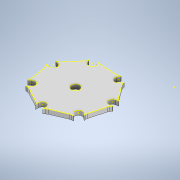
# Autodesk Inventor part: sprocket7_mk2
Saved by Autodesk Inventor 2020 (Build 240168000, 168)
## iProperties
Created: 2019-07-16
Part Number: sprocket7_mk2
Material: Generic
Document SubType Name: Modeling
Designer: erwin
Density: 1 g/cm^3
Appearance: Default
Author: erwin
Autodesk Inventor part; units mm, degrees
ref_plane "YZ Plane" through (0, 0, 0) normal (1, 0, 0) x (0, 1, 0)
ref_plane "XZ Plane" through (0, 0, 0) normal (0, 1, 0) x (-1, 0, 0)
ref_plane "XY Plane" through (0, 0, 0) normal (0, 0, 1) x (1, 0, 0)
sketch "Sketch2" plane through (0, 0, 0) normal (0, 1, 0) x (-1, 0, 0)
  line L0 (77.8598, 129.5505) -> (181.2412, 129.5505)
  line L1 (129.5505, 77.8598) -> (129.5505, 181.2412)
  line L2 (208.1814, 165.1629) -> (207.9893, 170.0518)
  line L3 (207.9893, 170.0518) -> (209.1581, 174.8028)
  line L4 (209.1581, 174.8028) -> (211.5965, 179.0445)
  line L5 (211.5965, 179.0445) -> (215.1139, 182.4454)
  line L6 (215.1139, 182.4454) -> (217.4859, 184.4007)
  line L7 (217.4859, 184.4007) -> (218.8706, 185.7147)
  line L8 (218.8706, 185.7147) -> (219.868, 187.3423)
  line L9 (219.868, 187.3423) -> (220.4102, 189.1727)
  line L10 (220.4102, 189.1727) -> (220.4602, 191.0809)
  line L11 (220.4602, 191.0809) -> (220.0145, 192.9371)
  line L12 (220.0145, 192.9371) -> (219.1037, 194.6147)
  line L13 (219.1037, 194.6147) -> (217.7897, 195.9994)
  line L14 (217.7897, 195.9994) -> (216.162, 196.9968)
  line L15 (216.162, 196.9968) -> (214.3317, 197.5389)
  line L16 (214.3317, 197.5389) -> (212.4235, 197.5889)
  line L17 (212.4235, 197.5889) -> (210.5673, 197.1433)
  line L18 (210.5673, 197.1433) -> (208.8897, 196.2324)
  line L19 (208.8897, 196.2324) -> (206.2971, 194.5807)
  line L20 (206.2971, 194.5807) -> (201.9757, 192.2864)
  line L21 (201.9757, 192.2864) -> (197.1881, 191.2781)
  line L22 (197.1881, 191.2781) -> (192.3084, 191.6346)
  line L23 (192.3084, 191.6346) -> (187.7182, 193.3281)
  line L24 (187.7182, 193.3281) -> (150.7331, 213.2305)
  line L25 (150.7331, 213.2305) -> (146.7911, 216.1285)
  line L26 (146.7911, 216.1285) -> (143.8054, 220.0046)
  line L27 (143.8054, 220.0046) -> (142.0094, 224.5557)
  line L28 (142.0094, 224.5557) -> (141.5435, 229.4261)
  line L29 (141.5435, 229.4261) -> (141.4937, 232.4997)
  line L30 (141.4937, 232.4997) -> (141.3297, 234.4016)
  line L31 (141.3297, 234.4016) -> (140.6791, 236.1962)
  line L32 (140.6791, 236.1962) -> (139.5861, 237.7613)
  line L33 (139.5861, 237.7613) -> (138.1253, 238.9901)
  line L34 (138.1253, 238.9901) -> (136.3963, 239.799)
  line L35 (136.3963, 239.799) -> (134.5168, 240.1329)
  line L36 (134.5168, 240.1329) -> (132.6149, 239.9689)
  line L37 (132.6149, 239.9689) -> (130.8203, 239.3182)
  line L38 (130.8203, 239.3182) -> (129.2552, 238.2252)
  line L39 (129.2552, 238.2252) -> (128.0264, 236.7645)
  line L40 (128.0264, 236.7645) -> (127.2175, 235.0354)
  line L41 (127.2175, 235.0354) -> (126.8836, 233.1559)
  line L42 (126.8836, 233.1559) -> (126.5586, 230.0991)
  line L43 (126.5586, 230.0991) -> (125.658, 225.29)
  line L44 (125.658, 225.29) -> (123.4612, 220.9182)
  line L45 (123.4612, 220.9182) -> (120.1401, 217.3254)
  line L46 (120.1401, 217.3254) -> (115.9541, 214.7925)
  line L47 (115.9541, 214.7925) -> (77.334, 198.2854)
  line L48 (77.334, 198.2854) -> (72.6104, 197.0103)
  line L49 (72.6104, 197.0103) -> (67.7184, 197.0926)
  line L50 (67.7184, 197.0926) -> (63.0404, 198.526)
  line L51 (63.0404, 198.526) -> (58.9421, 201.1984)
  line L52 (58.9421, 201.1984) -> (56.508, 203.0759)
  line L53 (56.508, 203.0759) -> (54.9188, 204.1335)
  line L54 (54.9188, 204.1335) -> (53.1101, 204.7437)
  line L55 (53.1101, 204.7437) -> (51.205, 204.865)
  line L56 (51.205, 204.865) -> (49.3334, 204.4891)
  line L57 (49.3334, 204.4891) -> (47.623, 203.6416)
  line L58 (47.623, 203.6416) -> (46.1901, 202.3802)
  line L59 (46.1901, 202.3802) -> (45.1326, 200.7911)
  line L60 (45.1326, 200.7911) -> (44.5223, 198.9823)
  line L61 (44.5223, 198.9823) -> (44.401, 197.0772)
  line L62 (44.401, 197.0772) -> (44.777, 195.2057)
  line L63 (44.777, 195.2057) -> (45.6245, 193.4952)
  line L64 (45.6245, 193.4952) -> (46.8858, 192.0624)
  line L65 (46.8858, 192.0624) -> (49.073, 189.9023)
  line L66 (49.073, 189.9023) -> (52.2714, 186.1998)
  line L67 (52.2714, 186.1998) -> (54.3197, 181.7566)
  line L68 (54.3197, 181.7566) -> (55.058, 176.9199)
  line L69 (55.058, 176.9199) -> (54.4284, 172.0679)
  line L70 (54.4284, 172.0679) -> (43.2549, 131.5815)
  line L71 (43.2549, 131.5815) -> (41.3067, 127.0934)
  line L72 (41.3067, 127.0934) -> (38.1923, 123.3201)
  line L73 (38.1923, 123.3201) -> (34.1549, 120.5564)
  line L74 (34.1549, 120.5564) -> (29.5103, 119.0184)
  line L75 (29.5103, 119.0184) -> (26.5248, 118.2859)
  line L76 (26.5248, 118.2859) -> (24.7071, 117.7028)
  line L77 (24.7071, 117.7028) -> (23.1023, 116.6692)
  line L78 (23.1023, 116.6692) -> (21.8196, 115.2553)
  line L79 (21.8196, 115.2553) -> (20.9467, 113.5577)
  line L80 (20.9467, 113.5577) -> (20.5428, 111.692)
  line L81 (20.5428, 111.692) -> (20.6356, 109.7853)
  line L82 (20.6356, 109.7853) -> (21.2187, 107.9677)
  line L83 (21.2187, 107.9677) -> (22.2523, 106.3628)
  line L84 (22.2523, 106.3628) -> (23.6661, 105.0802)
  line L85 (23.6661, 105.0802) -> (25.3638, 104.2072)
  line L86 (25.3638, 104.2072) -> (27.2295, 103.8034)
  line L87 (27.2295, 103.8034) -> (29.1361, 103.8961)
  line L88 (29.1361, 103.8961) -> (32.1886, 104.2594)
  line L89 (32.1886, 104.2594) -> (37.0775, 104.4515)
  line L90 (37.0775, 104.4515) -> (41.8285, 103.2827)
  line L91 (41.8285, 103.2827) -> (46.0703, 100.8443)
  line L92 (46.0703, 100.8443) -> (49.4712, 97.3269)
  line L93 (49.4712, 97.3269) -> (74.1582, 63.3482)
  line L94 (74.1582, 63.3482) -> (76.4524, 59.0268)
  line L95 (76.4524, 59.0268) -> (77.4607, 54.2392)
  line L96 (77.4607, 54.2392) -> (77.1042, 49.3595)
  line L97 (77.1042, 49.3595) -> (75.4108, 44.7692)
  line L98 (75.4108, 44.7692) -> (74.122, 41.9784)
  line L99 (74.122, 41.9784) -> (73.4446, 40.1937)
  line L100 (73.4446, 40.1937) -> (73.2521, 38.2945)
  line L101 (73.2521, 38.2945) -> (73.5578, 36.4102)
  line L102 (73.5578, 36.4102) -> (74.3407, 34.6693)
  line L103 (74.3407, 34.6693) -> (75.5476, 33.1902)
  line L104 (75.5476, 33.1902) -> (77.0961, 32.074)
  line L105 (77.0961, 32.074) -> (78.8808, 31.3966)
  line L106 (78.8808, 31.3966) -> (80.78, 31.2041)
  line L107 (80.78, 31.2041) -> (82.6643, 31.5098)
  line L108 (82.6643, 31.5098) -> (84.4053, 32.2927)
  line L109 (84.4053, 32.2927) -> (85.8843, 33.4996)
  line L110 (85.8843, 33.4996) -> (87.0006, 35.0481)
  line L111 (87.0006, 35.0481) -> (88.6197, 37.6612)
  line L112 (88.6197, 37.6612) -> (91.5177, 41.6033)
  line L113 (91.5177, 41.6033) -> (95.3937, 44.589)
  line L114 (95.3937, 44.589) -> (99.9449, 46.385)
  line L115 (99.9449, 46.385) -> (104.8153, 46.8509)
  line L116 (104.8153, 46.8509) -> (146.773, 44.9666)
  line L117 (146.773, 44.9666) -> (151.582, 44.066)
  line L118 (151.582, 44.066) -> (155.9538, 41.8692)
  line L119 (155.9538, 41.8692) -> (159.5466, 38.5481)
  line L120 (159.5466, 38.5481) -> (162.0796, 34.3621)
  line L121 (162.0796, 34.3621) -> (163.458, 31.6144)
  line L122 (163.458, 31.6144) -> (164.431, 29.9721)
  line L123 (164.431, 29.9721) -> (165.7958, 28.6375)
  line L124 (165.7958, 28.6375) -> (167.4596, 27.7016)
  line L125 (167.4596, 27.7016) -> (169.3089, 27.2283)
  line L126 (169.3089, 27.2283) -> (171.2177, 27.2497)
  line L127 (171.2177, 27.2497) -> (173.0559, 27.7644)
  line L128 (173.0559, 27.7644) -> (174.6983, 28.7374)
  line L129 (174.6983, 28.7374) -> (176.0329, 30.1023)
  line L130 (176.0329, 30.1023) -> (176.9687, 31.766)
  line L131 (176.9687, 31.766) -> (177.4421, 33.6153)
  line L132 (177.4421, 33.6153) -> (177.4207, 35.5241)
  line L133 (177.4207, 35.5241) -> (176.9059, 37.3624)
  line L134 (176.9059, 37.3624) -> (175.8725, 40.2575)
  line L135 (175.8725, 40.2575) -> (174.5974, 44.9811)
  line L136 (174.5974, 44.9811) -> (174.6797, 49.873)
  line L137 (174.6797, 49.873) -> (176.1131, 54.551)
  line L138 (176.1131, 54.551) -> (178.7855, 58.6494)
  line L139 (178.7855, 58.6494) -> (206.4189, 90.2784)
  line L140 (206.4189, 90.2784) -> (210.1214, 93.4767)
  line L141 (210.1214, 93.4767) -> (214.5647, 95.5251)
  line L142 (214.5647, 95.5251) -> (219.4013, 96.2633)
  line L143 (219.4013, 96.2633) -> (224.2533, 95.6338)
  line L144 (224.2533, 95.6338) -> (227.261, 94.9983)
  line L145 (227.261, 94.9983) -> (229.1516, 94.735)
  line L146 (229.1516, 94.735) -> (231.046, 94.97)
  line L147 (231.046, 94.97) -> (232.8151, 95.6873)
  line L148 (232.8151, 95.6873) -> (234.3382, 96.838)
  line L149 (234.3382, 96.838) -> (235.5115, 98.3438)
  line L150 (235.5115, 98.3438) -> (236.2552, 100.1018)
  line L151 (236.2552, 100.1018) -> (236.5185, 101.9925)
  line L152 (236.5185, 101.9925) -> (236.2835, 103.8869)
  line L153 (236.2835, 103.8869) -> (235.5662, 105.656)
  line L154 (235.5662, 105.656) -> (234.4155, 107.1791)
  line L155 (234.4155, 107.1791) -> (232.9098, 108.3524)
  line L156 (232.9098, 108.3524) -> (231.1517, 109.0961)
  line L157 (231.1517, 109.0961) -> (228.2439, 110.0932)
  line L158 (228.2439, 110.0932) -> (223.7558, 112.0414)
  line L159 (223.7558, 112.0414) -> (219.9824, 115.1559)
  line L160 (219.9824, 115.1559) -> (217.2187, 119.1932)
  line L161 (217.2187, 119.1932) -> (215.6807, 123.8378)
  line L162 (215.6807, 123.8378) -> (208.1814, 165.1629)
  circle A0 centre (129.5505, 129.5505) radius 10.75
  dimension "d0" = 21.5
  constraints: 326 end point, 1 centre point, 1 midpoint
  measures "d0" diameter of A0
extrude "Extrusion1" add sketch "Sketch2" along normal blind 12
sketch "Sketch3" plane through (0, 12, 0) normal (0, 1, 0) x (1, 0, 0)
  line L0 (-29.1361, -103.8961) -> (-32.1886, -104.2594)
  line L1 (-32.1886, -104.2594) -> (-37.0775, -104.4515)
  line L2 (-37.0775, -104.4515) -> (-41.8285, -103.2827)
  line L3 (-41.8285, -103.2827) -> (-46.0703, -100.8443)
  line L4 (-46.0703, -100.8443) -> (-49.4712, -97.3269)
  line L5 (-49.4712, -97.3269) -> (-74.1582, -63.3482)
  line L6 (-74.1582, -63.3482) -> (-76.4524, -59.0268)
  line L7 (-76.4524, -59.0268) -> (-77.4607, -54.2392)
  line L8 (-77.4607, -54.2392) -> (-77.1042, -49.3595)
  line L9 (-77.1042, -49.3595) -> (-75.4108, -44.7692)
  line L10 (-75.4108, -44.7692) -> (-74.122, -41.9784)
  line L11 (-74.122, -41.9784) -> (-73.4446, -40.1937)
  line L12 (-73.4446, -40.1937) -> (-73.2521, -38.2945)
  line L13 (-73.2521, -38.2945) -> (-73.5578, -36.4102)
  line L14 (-73.5578, -36.4102) -> (-74.3407, -34.6693)
  line L15 (-74.3407, -34.6693) -> (-75.5476, -33.1902)
  line L16 (-75.5476, -33.1902) -> (-77.0961, -32.074)
  line L17 (-77.0961, -32.074) -> (-78.8808, -31.3966)
  line L18 (-78.8808, -31.3966) -> (-80.78, -31.2041)
  line L19 (-80.78, -31.2041) -> (-82.6643, -31.5098)
  line L20 (-82.6643, -31.5098) -> (-84.4053, -32.2928)
  line L21 (-84.4053, -32.2928) -> (-85.8843, -33.4996)
  line L22 (-85.8843, -33.4996) -> (-87.0006, -35.0482)
  line L23 (-87.0006, -35.0482) -> (-88.6197, -37.6612)
  line L24 (-88.6197, -37.6612) -> (-91.5177, -41.6033)
  line L25 (-91.5177, -41.6033) -> (-95.3937, -44.589)
  line L26 (-95.3937, -44.589) -> (-99.9449, -46.385)
  line L27 (-99.9449, -46.385) -> (-104.8153, -46.8509)
  line L28 (-104.8153, -46.8509) -> (-146.773, -44.9666)
  line L29 (-146.773, -44.9666) -> (-151.582, -44.0659)
  line L30 (-151.582, -44.0659) -> (-155.9538, -41.8692)
  line L31 (-155.9538, -41.8692) -> (-159.5466, -38.5481)
  line L32 (-159.5466, -38.5481) -> (-162.0796, -34.3621)
  line L33 (-162.0796, -34.3621) -> (-163.458, -31.6144)
  line L34 (-163.458, -31.6144) -> (-164.431, -29.9721)
  line L35 (-164.431, -29.9721) -> (-165.7958, -28.6375)
  line L36 (-165.7958, -28.6375) -> (-167.4596, -27.7016)
  line L37 (-167.4596, -27.7016) -> (-169.3089, -27.2283)
  line L38 (-169.3089, -27.2283) -> (-171.2177, -27.2497)
  line L39 (-171.2177, -27.2497) -> (-173.0559, -27.7644)
  line L40 (-173.0559, -27.7644) -> (-174.6983, -28.7374)
  line L41 (-174.6983, -28.7374) -> (-176.0329, -30.1023)
  line L42 (-176.0329, -30.1023) -> (-176.9687, -31.766)
  line L43 (-176.9687, -31.766) -> (-177.4421, -33.6153)
  line L44 (-177.4421, -33.6153) -> (-177.4207, -35.5241)
  line L45 (-177.4207, -35.5241) -> (-176.9059, -37.3624)
  line L46 (-176.9059, -37.3624) -> (-175.8725, -40.2575)
  line L47 (-175.8725, -40.2575) -> (-174.5974, -44.9811)
  line L48 (-174.5974, -44.9811) -> (-174.6797, -49.873)
  line L49 (-174.6797, -49.873) -> (-176.1131, -54.551)
  line L50 (-176.1131, -54.551) -> (-178.7855, -58.6494)
  line L51 (-178.7855, -58.6494) -> (-206.4189, -90.2784)
  line L52 (-206.4189, -90.2784) -> (-210.1214, -93.4767)
  line L53 (-210.1214, -93.4767) -> (-214.5647, -95.5251)
  line L54 (-214.5647, -95.5251) -> (-219.4013, -96.2633)
  line L55 (-219.4013, -96.2633) -> (-224.2533, -95.6338)
  line L56 (-224.2533, -95.6338) -> (-227.261, -94.9983)
  line L57 (-227.261, -94.9983) -> (-229.1516, -94.735)
  line L58 (-229.1516, -94.735) -> (-231.046, -94.97)
  line L59 (-231.046, -94.97) -> (-232.8151, -95.6873)
  line L60 (-232.8151, -95.6873) -> (-234.3382, -96.838)
  line L61 (-234.3382, -96.838) -> (-235.5115, -98.3438)
  line L62 (-235.5115, -98.3438) -> (-236.2552, -100.1018)
  line L63 (-236.2552, -100.1018) -> (-236.5185, -101.9925)
  line L64 (-236.5185, -101.9925) -> (-236.2835, -103.8869)
  line L65 (-236.2835, -103.8869) -> (-235.5662, -105.656)
  line L66 (-235.5662, -105.656) -> (-234.4155, -107.1791)
  line L67 (-234.4155, -107.1791) -> (-232.9098, -108.3524)
  line L68 (-232.9098, -108.3524) -> (-231.1517, -109.0961)
  line L69 (-231.1517, -109.0961) -> (-228.2439, -110.0932)
  line L70 (-228.2439, -110.0932) -> (-223.7558, -112.0414)
  line L71 (-223.7558, -112.0414) -> (-219.9824, -115.1559)
  line L72 (-219.9824, -115.1559) -> (-217.2187, -119.1932)
  line L73 (-217.2187, -119.1932) -> (-215.6807, -123.8378)
  line L74 (-215.6807, -123.8378) -> (-208.1814, -165.1629)
  line L75 (-208.1814, -165.1629) -> (-207.9893, -170.0518)
  line L76 (-207.9893, -170.0518) -> (-209.1581, -174.8028)
  line L77 (-209.1581, -174.8028) -> (-211.5965, -179.0445)
  line L78 (-211.5965, -179.0445) -> (-215.1139, -182.4454)
  line L79 (-215.1139, -182.4454) -> (-217.4859, -184.4007)
  line L80 (-217.4859, -184.4007) -> (-218.8706, -185.7147)
  line L81 (-218.8706, -185.7147) -> (-219.868, -187.3423)
  line L82 (-219.868, -187.3423) -> (-220.4102, -189.1727)
  line L83 (-220.4102, -189.1727) -> (-220.4602, -191.0809)
  line L84 (-220.4602, -191.0809) -> (-220.0145, -192.9371)
  line L85 (-220.0145, -192.9371) -> (-219.1037, -194.6147)
  line L86 (-219.1037, -194.6147) -> (-217.7897, -195.9994)
  line L87 (-217.7897, -195.9994) -> (-216.162, -196.9968)
  line L88 (-216.162, -196.9968) -> (-214.3317, -197.5389)
  line L89 (-214.3317, -197.5389) -> (-212.4235, -197.5889)
  line L90 (-212.4235, -197.5889) -> (-210.5673, -197.1433)
  line L91 (-210.5673, -197.1433) -> (-208.8897, -196.2324)
  line L92 (-208.8897, -196.2324) -> (-206.2971, -194.5807)
  line L93 (-206.2971, -194.5807) -> (-201.9757, -192.2864)
  line L94 (-201.9757, -192.2864) -> (-197.1881, -191.2781)
  line L95 (-197.1881, -191.2781) -> (-192.3084, -191.6346)
  line L96 (-192.3084, -191.6346) -> (-187.7182, -193.3281)
  line L97 (-187.7182, -193.3281) -> (-150.7331, -213.2305)
  line L98 (-150.7331, -213.2305) -> (-146.7911, -216.1285)
  line L99 (-146.7911, -216.1285) -> (-143.8054, -220.0046)
  line L100 (-143.8054, -220.0046) -> (-142.0094, -224.5557)
  line L101 (-142.0094, -224.5557) -> (-141.5435, -229.4261)
  line L102 (-141.5435, -229.4261) -> (-141.4937, -232.4997)
  line L103 (-141.4937, -232.4997) -> (-141.3297, -234.4016)
  line L104 (-141.3297, -234.4016) -> (-140.6791, -236.1962)
  line L105 (-140.6791, -236.1962) -> (-139.5861, -237.7613)
  line L106 (-139.5861, -237.7613) -> (-138.1253, -238.9901)
  line L107 (-138.1253, -238.9901) -> (-136.3963, -239.799)
  line L108 (-136.3963, -239.799) -> (-134.5168, -240.1329)
  line L109 (-134.5168, -240.1329) -> (-132.6149, -239.9689)
  line L110 (-132.6149, -239.9689) -> (-130.8203, -239.3182)
  line L111 (-130.8203, -239.3182) -> (-129.2552, -238.2252)
  line L112 (-129.2552, -238.2252) -> (-128.0264, -236.7645)
  line L113 (-128.0264, -236.7645) -> (-127.2175, -235.0354)
  line L114 (-127.2175, -235.0354) -> (-126.8836, -233.1559)
  line L115 (-126.8836, -233.1559) -> (-126.5586, -230.0991)
  line L116 (-126.5586, -230.0991) -> (-125.658, -225.29)
  line L117 (-125.658, -225.29) -> (-123.4612, -220.9182)
  line L118 (-123.4612, -220.9182) -> (-120.1401, -217.3254)
  line L119 (-120.1401, -217.3254) -> (-115.9541, -214.7925)
  line L120 (-115.9541, -214.7925) -> (-77.334, -198.2854)
  line L121 (-77.334, -198.2854) -> (-72.6104, -197.0103)
  line L122 (-72.6104, -197.0103) -> (-67.7184, -197.0926)
  line L123 (-67.7184, -197.0926) -> (-63.0404, -198.526)
  line L124 (-63.0404, -198.526) -> (-58.9421, -201.1984)
  line L125 (-58.9421, -201.1984) -> (-56.508, -203.0759)
  line L126 (-56.508, -203.0759) -> (-54.9188, -204.1335)
  line L127 (-54.9188, -204.1335) -> (-53.1101, -204.7437)
  line L128 (-53.1101, -204.7437) -> (-51.205, -204.865)
  line L129 (-51.205, -204.865) -> (-49.3334, -204.4891)
  line L130 (-49.3334, -204.4891) -> (-47.623, -203.6416)
  line L131 (-47.623, -203.6416) -> (-46.1901, -202.3802)
  line L132 (-46.1901, -202.3802) -> (-45.1326, -200.7911)
  line L133 (-45.1326, -200.7911) -> (-44.5223, -198.9823)
  line L134 (-44.5223, -198.9823) -> (-44.401, -197.0772)
  line L135 (-44.401, -197.0772) -> (-44.777, -195.2057)
  line L136 (-44.777, -195.2057) -> (-45.6245, -193.4952)
  line L137 (-45.6245, -193.4952) -> (-46.8858, -192.0624)
  line L138 (-46.8858, -192.0624) -> (-49.073, -189.9023)
  line L139 (-49.073, -189.9023) -> (-52.2714, -186.1998)
  line L140 (-52.2714, -186.1998) -> (-54.3197, -181.7566)
  line L141 (-54.3197, -181.7566) -> (-55.058, -176.9199)
  line L142 (-55.058, -176.9199) -> (-54.4284, -172.0679)
  line L143 (-54.4284, -172.0679) -> (-43.2549, -131.5815)
  line L144 (-43.2549, -131.5815) -> (-41.3067, -127.0934)
  line L145 (-41.3067, -127.0934) -> (-38.1923, -123.3201)
  line L146 (-38.1923, -123.3201) -> (-34.1549, -120.5564)
  line L147 (-34.1549, -120.5564) -> (-29.5103, -119.0184)
  line L148 (-29.5103, -119.0184) -> (-26.5248, -118.2859)
  line L149 (-26.5248, -118.2859) -> (-24.7071, -117.7028)
  line L150 (-24.7071, -117.7028) -> (-23.1022, -116.6692)
  line L151 (-23.1022, -116.6692) -> (-21.8196, -115.2553)
  line L152 (-21.8196, -115.2553) -> (-20.9466, -113.5577)
  line L153 (-20.9466, -113.5577) -> (-20.5428, -111.692)
  line L154 (-20.5428, -111.692) -> (-20.6356, -109.7853)
  line L155 (-20.6356, -109.7853) -> (-21.2186, -107.9677)
  line L156 (-21.2186, -107.9677) -> (-22.2523, -106.3628)
  line L157 (-22.2523, -106.3628) -> (-23.6661, -105.0802)
  line L158 (-23.6661, -105.0802) -> (-25.3638, -104.2072)
  line L159 (-25.3638, -104.2072) -> (-27.2295, -103.8034)
  line L160 (-27.2295, -103.8034) -> (-29.1361, -103.8961)
  circle A0 centre (-129.5505, -129.5505) radius 10.75
  circle A1 centre (-80.5613, -38.5133) radius 7.2498
  line L161 (-129.5505, -129.5505) -> (-80.5613, -38.5133) construction
  line L162 (-80.5613, -38.5133) -> (-90.0386, -56.1252) construction
  line L163 (-89.3672, -33.7746) -> (-98.8446, -51.3865)
  line L164 (-81.2327, -60.8639) -> (-71.7553, -43.252)
  arc A2 (-71.7553, -43.252) -> (-89.3672, -33.7746) centre (-80.5613, -38.5133) ccw
  arc A3 (-98.8446, -51.3865) -> (-81.2327, -60.8639) centre (-90.0386, -56.1252) ccw
  circle A4 centre (-170.182, -34.4884) radius 7.2498
  arc A5 (-160.9867, -30.5581) -> (-179.3773, -38.4186) centre (-170.182, -34.4884) ccw
  line L165 (-170.182, -34.4884) -> (-162.3215, -52.879) construction
  line L166 (-179.3773, -38.4186) -> (-171.5168, -56.8092)
  line L167 (-153.1262, -48.9487) -> (-160.9867, -30.5581)
  arc A6 (-171.5168, -56.8092) -> (-153.1262, -48.9487) centre (-162.3215, -52.879) ccw
  circle A7 centre (-229.2063, -102.0472) radius 7.2498
  arc A8 (-226.546, -92.4076) -> (-231.8667, -111.6869) centre (-229.2063, -102.0472) ccw
  line L168 (-229.2063, -102.0472) -> (-209.9271, -107.368) construction
  line L169 (-231.8667, -111.6869) -> (-212.5875, -117.0076)
  line L170 (-207.2667, -97.7283) -> (-226.546, -92.4076)
  arc A9 (-212.5875, -117.0076) -> (-207.2667, -97.7283) centre (-209.9271, -107.368) ccw
  circle A10 centre (-213.1878, -190.3166) radius 7.2498
  arc A11 (-219.0657, -182.2264) -> (-207.31, -198.4067) centre (-213.1878, -190.3166) ccw
  line L171 (-213.1878, -190.3166) -> (-197.0075, -178.5609) construction
  line L172 (-207.31, -198.4067) -> (-191.1296, -186.651)
  line L173 (-202.8853, -170.4707) -> (-219.0657, -182.2264)
  arc A12 (-191.1296, -186.651) -> (-202.8853, -170.4707) centre (-197.0075, -178.5609) ccw
  circle A13 centre (-134.1887, -232.8278) radius 7.2498
  arc A14 (-144.1786, -232.3792) -> (-124.1987, -233.2765) centre (-134.1887, -232.8278) ccw
  line L174 (-134.1887, -232.8278) -> (-133.2914, -212.848) construction
  line L175 (-124.1987, -233.2765) -> (-123.3015, -213.2966)
  line L176 (-143.2813, -212.3993) -> (-144.1786, -232.3792)
  arc A15 (-123.3015, -213.2966) -> (-143.2813, -212.3993) centre (-133.2914, -212.848) ccw
  circle A16 centre (-51.6969, -197.5691) radius 7.2498
  arc A17 (-58.2763, -205.0998) -> (-45.1175, -190.0384) centre (-51.6969, -197.5691) ccw
  line L177 (-51.6969, -197.5691) -> (-66.7583, -184.4104) construction
  line L178 (-45.1175, -190.0384) -> (-60.1789, -176.8796)
  line L179 (-73.3377, -191.9411) -> (-58.2763, -205.0998)
  arc A18 (-60.1789, -176.8796) -> (-73.3377, -191.9411) centre (-66.7583, -184.4104) ccw
  circle A19 centre (-27.8304, -111.091) radius 7.2498
  arc A20 (-26.0449, -120.9303) -> (-29.616, -101.2517) centre (-27.8304, -111.091) ccw
  line L180 (-27.8304, -111.091) -> (-47.509, -114.6622) construction
  line L181 (-29.616, -101.2517) -> (-49.2946, -104.8229)
  line L182 (-45.7235, -124.5015) -> (-26.0449, -120.9303)
  arc A21 (-49.2946, -104.8229) -> (-45.7235, -124.5015) centre (-47.509, -114.6622) ccw
  point P0 (0, 0)
  point P1 (-85.3, -47.3192)
  point P2 (-166.2517, -43.6837)
  point P3 (-219.5667, -104.7076)
  point P4 (-205.0977, -184.4387)
  point P5 (-133.74, -222.8379)
  point P6 (-59.2276, -190.9897)
  point P7 (-37.6697, -112.8766)
  point P8 (-141.4117, -233.4507)
  point P9 (-127.0505, -234.0956)
  point P10 (-123.6617, -221.3171)
  point P11 (-143.6415, -220.4198)
  point P12 (-55.7134, -203.6047)
  point P13 (-46.2551, -192.7788)
  point P14 (-54.1328, -182.162)
  point P15 (-67.2916, -197.2234)
  point P16 (-25.6159, -117.9944)
  point P17 (-26.2966, -104.0053)
  point P18 (-41.3951, -103.3893)
  point P19 (-37.8239, -123.0679)
  point P20 (-73.7833, -41.0861)
  point P21 (-86.4424, -34.2739)
  point P22 (-95.0401, -44.3166)
  point P23 (-77.4282, -53.7939)
  point P24 (-174.6722, -49.4267)
  point P25 (-156.2816, -41.5662)
  point P26 (-163.9445, -30.7933)
  point P27 (-177.1633, -36.4432)
  point P28 (-232.0308, -108.7243)
  point P29 (-220.3267, -114.8717)
  point P30 (-215.006, -95.5924)
  point P31 (-230.0989, -94.8525)
  point P32 (-218.1783, -185.0577)
  point P33 (-209.7285, -196.6879)
  point P34 (-197.6249, -191.3701)
  point P35 (-209.3806, -175.1898)
  dimension "d3" = 20
  dimension "d4" = 20
  dimension "d7" = 360
  constraints: 58 end point, 28 point on circle, 21 centre point, 7 tangent, 1 midpoint, 1 parallel, 1 point on line, 92 other
  measures "d3" diameter of A3
  measures "d4" distance of L162.end L161.end
extrude "Extrusion2" cut sketch "Sketch3" against normal through all contours L160 A19 L149 L148 L147 L146 L182 A21 L181 L2 L1 L0 | L0 L1 L2 L181 A20 L182 L146 L147 L148 L149 L150 L151 L152 L153 L154 L155 L156 L157 L158 L159 L160 | L160 L159 A19 | A19 | L159 L158 A19 | A19 L150 L149 | L158 L157 A19 | A19 L151 L150 | L157 L156 A19 | A19 L152 L151 | L156 L155 A19 | A19 L153 L152 | L155 L154 A19 | A19 L154 L153 | L164 A3 L163 L25 L24 L23 L22 A1 L11 L10 L9 L8 | L8 L9 L10 L11 L12 L13 L14 L15 L16 L17 L18 L19 L20 L21 L22 L23 L24 L25 L163 A2 L164 | L178 A17 L179 L123 L124 L125 L126 L127 L128 L129 L130 L131 L132 L133 L134 L135 L136 L137 L138 L139 L140 | L140 L139 L138 L137 A16 L126 L125 L124 L123 L179 A18 L178 | A1 L12 L11 | A1 | L22 L21 A1 | A1 L13 L12 | L21 L20 A1 | L20 L19 A1 | A1 L14 L13 | L137 L136 A16 | A16 | L19 L18 A1 | A1 L15 L14 | L136 L135 A16 | A16 L127 L126 | L18 L17 A1 | A1 L16 L15 | L135 L134 A16 | A16 L128 L127 | L17 L16 A1 | L167 A6 L166 L48 L47 L46 L45 A4 L34 L33 L32 L31 | L31 L32 L33 L34 L35 L36 L37 L38 L39 L40 L41 L42 L43 L44 L45 L46 L47 L48 L166 A5 L167 | A16 L129 L128 | L134 L133 A16 | A16 L130 L129 | L133 L132 A16 | A16 L131 L130 | L132 L131 A16 | L175 A14 L176 L100 L101 L102 L103 L104 L105 L106 L107 L108 L109 L110 L111 L112 L113 L114 L115 L116 L117 | L117 L116 L115 L114 A13 L103 L102 L101 L100 L176 A15 L175 | A4 L35 L34 | A4 | A4 L36 L35 | L45 L44 A4 | A4 L37 L36 | L44 L43 A4 | A4 L38 L37 | L114 L113 A13 | A13 | L43 L42 A4 | A4 L39 L38 | L113 L112 A13 | L42 L41 A4 | A4 L40 L39 | L112 L111 A13 | A13 L104 L103 | L41 L40 A4 | L170 A9 L169 L71 L70 L69 L68 A7 L57 L56 L55 L54 | L54 L55 L56 L57 L58 L59 L60 L61 L62 L63 L64 L65 L66 L67 L68 L69 L70 L71 L169 A8 L170 | L111 L110 A13 | A13 L105 L104 | L110 L109 A13 | A13 L106 L105 | L109 L108 A13 | A13 L107 L106 | L108 L107 A13 | L172 A11 L173 L77 L78 L79 L80 L81 L82 L83 L84 L85 L86 L87 L88 L89 L90 L91 L92 L93 L94 | L94 L93 L92 L91 A10 L80 L79 L78 L77 L173 A12 L172 | A7 L58 L57 | A7 | A7 L59 L58 | L68 L67 A7 | A7 L60 L59 | L67 L66 A7 | A7 L61 L60 | L91 L90 A10 | A10 | L66 L65 A7 | A7 L62 L61 | L90 L89 A10 | L65 L64 A7 | A7 L63 L62 | L89 L88 A10 | A10 L81 L80 | L64 L63 A7 | L88 L87 A10 | A10 L82 L81 | L87 L86 A10 | A10 L83 L82 | L86 L85 A10 | A10 L84 L83 | L85 L84 A10
sketch "Sketch4" plane through (0, 12, 0) normal (0, 1, 0) x (1, 0, 0)
  line L0 (-98.8446, -51.3865) -> (-95.0401, -44.3166) projected
  line L1 (-95.0401, -44.3166) -> (-95.3937, -44.589) projected
  line L2 (-95.3937, -44.589) -> (-99.9449, -46.385) projected
  line L3 (-99.9449, -46.385) -> (-104.8153, -46.8509) projected
  line L4 (-104.8153, -46.8509) -> (-146.773, -44.9666) projected
  line L5 (-146.773, -44.9666) -> (-151.582, -44.0659) projected
  line L6 (-151.582, -44.0659) -> (-155.9538, -41.8692) projected
  line L7 (-155.9538, -41.8692) -> (-156.2816, -41.5662) projected
  line L8 (-156.2816, -41.5662) -> (-153.1262, -48.9487) projected
  arc A0 (-171.5168, -56.8092) -> (-153.1262, -48.9487) centre (-162.3215, -52.879) ccw projected
  line L9 (-171.5168, -56.8092) -> (-174.6722, -49.4267) projected
  line L10 (-174.6722, -49.4267) -> (-174.6797, -49.873) projected
  line L11 (-174.6797, -49.873) -> (-176.1131, -54.551) projected
  line L12 (-176.1131, -54.551) -> (-178.7855, -58.6494) projected
  line L13 (-178.7855, -58.6494) -> (-206.4189, -90.2784) projected
  line L14 (-206.4189, -90.2784) -> (-210.1214, -93.4767) projected
  line L15 (-210.1214, -93.4767) -> (-214.5647, -95.5251) projected
  line L16 (-214.5647, -95.5251) -> (-215.006, -95.5924) projected
  line L17 (-215.006, -95.5924) -> (-207.2667, -97.7283) projected
  arc A1 (-212.5875, -117.0076) -> (-207.2667, -97.7283) centre (-209.9271, -107.368) ccw projected
  line L18 (-212.5875, -117.0076) -> (-220.3267, -114.8717) projected
  line L19 (-220.3267, -114.8717) -> (-219.9824, -115.1559) projected
  line L20 (-219.9824, -115.1559) -> (-217.2187, -119.1932) projected
  line L21 (-217.2187, -119.1932) -> (-215.6807, -123.8378) projected
  line L22 (-215.6807, -123.8378) -> (-208.1814, -165.1629) projected
  line L23 (-208.1814, -165.1629) -> (-207.9893, -170.0518) projected
  line L24 (-207.9893, -170.0518) -> (-209.1581, -174.8028) projected
  line L25 (-209.1581, -174.8028) -> (-209.3806, -175.1898) projected
  line L26 (-209.3806, -175.1898) -> (-202.8853, -170.4707) projected
  arc A2 (-191.1296, -186.651) -> (-202.8853, -170.4707) centre (-197.0075, -178.5609) ccw projected
  line L27 (-191.1296, -186.651) -> (-197.6249, -191.3701) projected
  line L28 (-197.6249, -191.3701) -> (-197.1881, -191.2781) projected
  line L29 (-197.1881, -191.2781) -> (-192.3084, -191.6346) projected
  line L30 (-192.3084, -191.6346) -> (-187.7182, -193.3281) projected
  line L31 (-187.7182, -193.3281) -> (-150.7331, -213.2305) projected
  line L32 (-150.7331, -213.2305) -> (-146.7911, -216.1285) projected
  line L33 (-146.7911, -216.1285) -> (-143.8054, -220.0046) projected
  line L34 (-143.8054, -220.0046) -> (-143.6415, -220.4198) projected
  line L35 (-143.6415, -220.4198) -> (-143.2813, -212.3993) projected
  arc A3 (-123.3015, -213.2966) -> (-143.2813, -212.3993) centre (-133.2914, -212.848) ccw projected
  line L36 (-123.3015, -213.2966) -> (-123.6617, -221.3171) projected
  line L37 (-123.6617, -221.3171) -> (-123.4612, -220.9182) projected
  line L38 (-123.4612, -220.9182) -> (-120.1401, -217.3254) projected
  line L39 (-120.1401, -217.3254) -> (-115.9541, -214.7925) projected
  line L40 (-115.9541, -214.7925) -> (-77.334, -198.2854) projected
  line L41 (-77.334, -198.2854) -> (-72.6104, -197.0103) projected
  line L42 (-72.6104, -197.0103) -> (-67.7184, -197.0926) projected
  line L43 (-67.7184, -197.0926) -> (-67.2916, -197.2234) projected
  line L44 (-67.2916, -197.2234) -> (-73.3377, -191.9411) projected
  arc A4 (-60.1789, -176.8796) -> (-73.3377, -191.9411) centre (-66.7583, -184.4104) ccw projected
  line L45 (-60.1789, -176.8796) -> (-54.1328, -182.162) projected
  line L46 (-54.1328, -182.162) -> (-54.3197, -181.7566) projected
  line L47 (-54.3197, -181.7566) -> (-55.058, -176.9199) projected
  line L48 (-55.058, -176.9199) -> (-54.4284, -172.0679) projected
  line L49 (-54.4284, -172.0679) -> (-43.2549, -131.5815) projected
  line L50 (-43.2549, -131.5815) -> (-41.3067, -127.0934) projected
  line L51 (-41.3067, -127.0934) -> (-38.1923, -123.3201) projected
  line L52 (-38.1923, -123.3201) -> (-37.8239, -123.0679) projected
  line L53 (-37.8239, -123.0679) -> (-45.7235, -124.5015) projected
  arc A5 (-49.2946, -104.8229) -> (-45.7235, -124.5015) centre (-47.509, -114.6622) ccw projected
  line L54 (-49.2946, -104.8229) -> (-41.3951, -103.3893) projected
  line L55 (-41.3951, -103.3893) -> (-41.8285, -103.2827) projected
  line L56 (-41.8285, -103.2827) -> (-46.0703, -100.8443) projected
  line L57 (-46.0703, -100.8443) -> (-49.4712, -97.3269) projected
  line L58 (-49.4712, -97.3269) -> (-74.1582, -63.3482) projected
  line L59 (-74.1582, -63.3482) -> (-76.4524, -59.0268) projected
  line L60 (-76.4524, -59.0268) -> (-77.4607, -54.2392) projected
  line L61 (-77.4607, -54.2392) -> (-77.4282, -53.7939) projected
  line L62 (-77.4282, -53.7939) -> (-81.2327, -60.8639) projected
  arc A6 (-98.8446, -51.3865) -> (-81.2327, -60.8639) centre (-90.0386, -56.1252) ccw projected
  circle A7 centre (-129.5505, -129.5505) radius 10.75 projected
  point P0 (0, 0)
body "Solid1"
